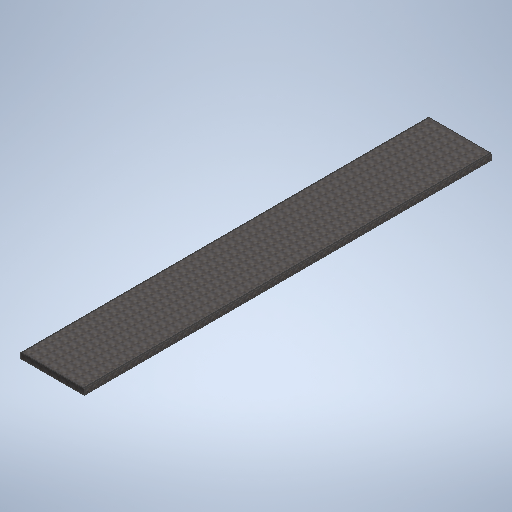
# Autodesk Inventor part: Concrete Walkway
Saved by Autodesk Inventor 2025 (Build 290162000, 162)
## iProperties
Created: 2024-06-26
Part Number: Concrete Walkway
Material: Concrete
Document SubType Name: Modeling
Designer: track
Density: 2.40731 g/cm^3
Appearance: Exposed Aggregate - Coarse
Author: track
Autodesk Inventor part; units mm, degrees
ref_plane "YZ Plane" through (0, 0, 0) normal (1, 0, 0) x (0, 1, 0)
ref_plane "XZ Plane" through (0, 0, 0) normal (0, 1, 0) x (-1, 0, 0)
ref_plane "XY Plane" through (0, 0, 0) normal (0, 0, 1) x (1, 0, 0)
sketch "Sketch1" plane through (0, 0, 0) normal (0, 0, 1) x (1, 0, 0)
  line L0 (838.2, -76.2) -> (-838.2, -76.2)
  line L1 (-838.2, -76.2) -> (-838.2, 76.2)
  line L2 (-838.2, 76.2) -> (838.2, 76.2)
  line L3 (838.2, 76.2) -> (838.2, -76.2)
  line L4 (838.2, -76.2) -> (-838.2, 76.2) construction
  line L5 (-838.2, -76.2) -> (838.2, 76.2) construction
  point P0 (0, 0)
  dimension "d0" = 152.4
  dimension "d1" = 1676.4
  constraints: 12 end point, 2 midpoint, 2 parallel, 1 horizontal, 1 perpendicular
  measures "d0" distance of L0.end L1.end
  measures "d1" distance of L1.end L2.end
extrude "Extrusion1" add sketch "Sketch1" against normal blind 10560.05
sketch "Sketch2" plane through (0, 0, 0) normal (0, 0, 1) x (1, 0, 0)
  line L0 (838.2, -76.2) -> (-838.2, -76.2) projected
  line L1 (825.5, -76.2) -> (825.5, 50.8)
  line L2 (825.5, 50.8) -> (800.1, 66.675)
  line L3 (800.1, 66.675) -> (800.1, 76.2)
  line L4 (-838.2, 76.2) -> (838.2, 76.2) projected
  line L5 (800.1, 76.2) -> (838.2, 76.2)
  line L6 (838.2, 76.2) -> (838.2, -76.2)
  line L7 (825.5, -76.2) -> (838.2, -76.2)
  line L8 (0, 76.2) -> (0, -76.2) construction
  line L9 (-838.2, -76.2) -> (838.2, -76.2)
  line L10 (-825.5, -76.2) -> (-825.5, 50.8)
  line L11 (-825.5, 50.8) -> (-800.1, 66.675)
  line L12 (-800.1, 66.675) -> (-800.1, 76.2)
  line L13 (838.2, 76.2) -> (-838.2, 76.2)
  line L14 (-800.1, 76.2) -> (-838.2, 76.2)
  line L15 (-838.2, 76.2) -> (-838.2, -76.2)
  line L16 (-825.5, -76.2) -> (-838.2, -76.2)
  point P0 (0, 0)
  dimension "d4" = 12.7
  dimension "d5" = 25.4
  dimension "d6" = 15.875
  dimension "d7" = 127
  constraints: 30 end point, 9 symmetric about line, 4 point on line, 2 midpoint, 2 vertical, 1 collinear, 1 horizontal, 1 perpendicular
  measures "d4" distance between parallel lines of L6 L1
  measures "d5" horizontal distance of L1.end L2.end
  measures "d6" vertical distance of L1.end L2.end
  measures "d7" distance of L1.start L1.end
extrude "Extrusion2" cut sketch "Sketch2" against normal through all contours L0 L1 L2 L3 L4 L6 | L0 L15 L4 L12 L11 L10
body "Solid1"
